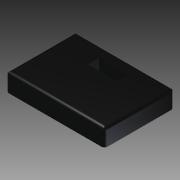
# Autodesk Inventor part: UB16NKG015F-NR
Saved by Autodesk Inventor 2015 SP1 (Build 190203100, 203)
## iProperties
Category: Electrical
Company: Autodesk Inc.
Created: 2014-12-16
Part Number: UB16NKG015F-NR
Catalog Web Link: http://www.nkkswitches.com/
Description: UB_ill_black_cap-Illuminated Pushbuttons - Series UB
Vendor: NKK Switches
Document SubType Name: Modeling
Designer: Autodesk Inc.
Manufacturer: NKKSWITCHES
Mass: 0.576302 g
Surface Area: 5.89123 cm^2
Volume: 0.576302 cm^3
Density: 1 g/cm^3
Material: Generic
Appearance: PSOLRGB-0-0-0
PSOL_IDENT_2: 06.2008 00:00:00},{VERSION=},{LINEID=10},{LINESUBID=-1},{WBVAR=MT}  {NB=UBNK-black_cap},{LINA=UBNK-b
PSOL_IDENT_3: lack_cap},{KT=DUMMY},{SRS=UB},{MT=NK},{WID=0.669},{WID2=0.604}
SUPPLIER: NKKSWITCHES
Title: UBNK-black_cap
Author: Autodesk Inc.
Comments: Illuminated Pushbuttons - Series UB
Autodesk Inventor part; units mm, degrees
sketch "Sketch_1" plane through (0, 0, 0) normal (0, 1, 0) x (-1, 0, 0)
  line L0 (8.4963, -5.4864) -> (8.4963, 5.4864)
  arc A0 (8.4963, 5.4864) -> (7.9883, 5.9944) centre (7.9883, 5.4864) ccw
  line L1 (7.9883, 5.9944) -> (-7.9883, 5.9944)
  arc A1 (-7.9883, 5.9944) -> (-8.4963, 5.4864) centre (-7.9883, 5.4864) ccw
  line L2 (-8.4963, 5.4864) -> (-8.4963, -5.4864)
  arc A2 (-8.4963, -5.4864) -> (-7.9883, -5.9944) centre (-7.9883, -5.4864) ccw
  line L3 (-7.9883, -5.9944) -> (7.9883, -5.9944)
  arc A3 (7.9883, -5.9944) -> (8.4963, -5.4864) centre (7.9883, -5.4864) ccw
  constraints: 8 end point, 8 point on circle, 4 centre point
extrude "Extrusion1" add sketch "Sketch_1" along normal blind 2.9972
sketch "Sketch_6" plane through (0, 0, 0) normal (0, 0, 1) x (1, 0, 0)
  line L0 (-10.16, 5.08) -> (-10.16, -2.54)
  line L1 (-10.16, -2.54) -> (10.16, -2.54)
  line L2 (10.16, -2.54) -> (10.16, 5.08)
  line L3 (10.16, 5.08) -> (-10.16, 5.08)
  line L4 (-8.4963, 0) -> (8.4963, 0)
  line L5 (8.4963, 0) -> (8.4963, 2.4892)
  arc A0 (8.4963, 2.4892) -> (7.9883, 2.9972) centre (7.9883, 2.4892) ccw
  line L6 (7.9883, 2.9972) -> (-7.9883, 2.9972)
  arc A1 (-7.9883, 2.9972) -> (-8.4963, 2.4892) centre (-7.9883, 2.4892) ccw
  line L7 (-8.4963, 2.4892) -> (-8.4963, 0)
  constraints: 16 end point, 4 point on circle, 2 centre point
extrude "Extrusion2" cut sketch "Sketch_6" along normal mid plane 15.24
sketch "Sketch_9" plane through (0, 0, 0) normal (1, 0, 0) x (0, 1, 0)
  line L0 (5.08, 10.16) -> (-2.54, 10.16)
  line L1 (-2.54, 10.16) -> (-2.54, -10.16)
  line L2 (-2.54, -10.16) -> (5.08, -10.16)
  line L3 (5.08, -10.16) -> (5.08, 10.16)
  line L4 (0, 5.9944) -> (0, -5.9944)
  line L5 (0, -5.9944) -> (2.4892, -5.9944)
  arc A0 (2.4892, -5.9944) -> (2.9972, -5.4864) centre (2.4892, -5.4864) ccw
  line L6 (2.9972, -5.4864) -> (2.9972, 5.4864)
  arc A1 (2.9972, 5.4864) -> (2.4892, 5.9944) centre (2.4892, 5.4864) ccw
  line L7 (2.4892, 5.9944) -> (0, 5.9944)
  constraints: 16 end point, 4 point on circle, 2 centre point
extrude "Extrusion3" cut sketch "Sketch_9" along normal mid plane 20.32
sketch "Sketch_4" plane through (-8.4963, 0, 0) normal (1, 0, 0) x (0, 0, -1)
  line L0 (-1.905, 0) -> (1.905, 0)
  line L1 (1.905, 0) -> (1.905, 1.016)
  line L2 (1.905, 1.016) -> (-1.905, 1.016)
  line L3 (-1.905, 1.016) -> (-1.905, 0)
  constraints: 8 end point
extrude "Extrusion4" cut sketch "Sketch_4" along normal blind 0.508
sketch "Sketch_5" plane through (0, 0, 0) normal (0, 1, 0) x (-1, 0, 0)
  line L0 (2.5019, -4.0513) -> (2.5019, -2.1463)
  line L1 (2.5019, -2.1463) -> (-2.5019, -2.1463)
  line L2 (-2.5019, -2.1463) -> (-2.5019, -4.0513)
  line L3 (-2.5019, -4.0513) -> (2.5019, -4.0513)
  constraints: 8 end point
extrude "Extrusion5" cut sketch "Sketch_5" along normal blind 5.08
ref_plane "P_XY" through (0, 0, 0) normal (0, 1, 0) x (1, 0, 0)
ref_plane "P_YZ" through (0, 0, 0) normal (1, 0, 0) x (0, 0, -1)
ref_plane "P_ZX" through (0, 0, 0) normal (0, 0, -1) x (0, 1, 0)
ref_plane "SPOT_XY" through (0, 0, -3.0988) normal (0, -1, 0) x (1, 0, 0)
ref_plane "SPOT_YZ" through (0, 0, -3.0988) normal (1, 0, 0) x (0, 0, 1)
ref_plane "SPOT_ZX" through (0, 0, -3.0988) normal (0, 0, 1) x (0, -1, 0)
body "Solid1"
